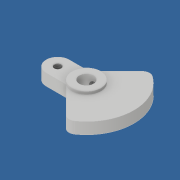
# Autodesk Inventor part: Kurbel 19
Saved by Autodesk Inventor 2018 (Build 220112000, 112)
## iProperties
Created: 2018-10-20
Part Number: Kurbel 19
Material: Generisch
Document SubType Name: Modeling
Designer: M.Knabel
Density: 1 g/cm^3
Appearance: Vorgabe
Mass: 1.78961 g
Surface Area: 14.1512 cm^2
Volume: 1.78961 cm^3
Author: M.Knabel
Autodesk Inventor part; units mm, degrees
ref_plane "YZ Plane" through (0, 0, 0) normal (1, 0, 0) x (0, 1, 0)
ref_plane "XZ Plane" through (0, 0, 0) normal (0, 1, 0) x (-1, 0, 0)
ref_plane "XY Plane" through (0, 0, 0) normal (0, 0, 1) x (1, 0, 0)
sketch "Skizze1" plane through (0, 0, 0) normal (0, 0, 1) x (1, 0, 0)
  line L0 (0, -20.5159) -> (0, 20.5159) projected
  line L1 (-20.1, 0) -> (22.6, 0) projected
  circle A0 centre (0, 0) radius 2.5
  arc A1 (-3, 4) -> (-3, -4) centre (0, 0) ccw
  arc A2 (7.5831, -14.6542) -> (7.5831, 14.6542) centre (0, 0) ccw
  line L2 (-3.5355, 3.5355) -> (7.5831, 14.6542)
  line L3 (-3.5355, -3.5355) -> (7.5831, -14.6542)
  line L4 (-3, 4) -> (-10, 4)
  line L5 (-3, -4) -> (-10, -4)
  arc A3 (-10, 4) -> (-10, -4) centre (-10, 0) ccw
  dimension "d0" = 5
  dimension "d1" = 10
  dimension "d3" = 33
  dimension "d4" = 90
  dimension "d5" = 4
  dimension "d6" = 10
  constraints: 8 end point, 8 point on circle, 4 centre point, 3 coincident, 3 tangent, 1 horizontal, 1 parallel, 1 point on line, 1 symmetric about line, 1 other
  measures "d0" diameter of A0
  measures "d1" diameter of A1
  measures "d3" diameter of A2
  measures "d4" angle of L3 L2
  measures "d5" radius of A3
  measures "d6" distance of A3.centre point (0, 0)
extrude "Extrusion1" add sketch "Skizze1" along normal blind 4 contours L3 L5 A1 L1 A0 L0 | L0 A0 L1 A2 L3 | L5 A3 L1 A1 L3 | L3 A1 L5 | L1 A1 L4 L2 L0 A0 | A0 L0 L2 A2 L1 | L1 A3 L4 L2 A1 | L2 L4 A1
fillet "Rundung1" radius 2.5 2 edges at (7.5831, 14.6542, 2) (7.5831, -14.6542, 2)
sketch "Skizze2" plane through (0, 0, 4) normal (0, 0, 1) x (1, 0, 0)
  arc A0 (-10, 4) -> (-10, -4) centre (-10, 0) ccw projected
  line L0 (0, -20.5159) -> (0, 20.5159) projected
  point P0 (0, 0)
  constraints: 1 coincident
hole "Bohrung1" at (-10, 0, 4) direction (0, 0, -1) diameter 2.459 end through all thread size "M3x0.5" class "6H" standard "ISO Metric profile"
sketch "Skizze3" plane through (0, 0, 4) normal (0, 0, 1) x (1, 0, 0)
  line L0 (0, -20.5159) -> (0, 20.5159) projected
  line L1 (-20.1, 0) -> (22.6, 0) projected
  line L2 (-10, -4) -> (-3.0711, -4) projected
  circle A0 centre (0, 0) radius 5.043
  circle A1 centre (0, 0) radius 2.5
  dimension "d17" = 5
  constraints: 2 coincident, 1 centre point, 3 other
  measures "d17" diameter of A1
extrude "Extrusion2" add sketch "Skizze3" along normal blind 1 contours A0 L1 A1 L0 | L0 A1 L1 A0 | L1 A1 L0 A0 | L1 A0 L0 A1
ref_plane "Arbeitsebene1" through (0, 10, 0) normal (0, 1, 0) x (-1, 0, 0)
sketch "Skizze7" plane through (0, 10, 0) normal (0, 1, 0) x (-1, 0, 0)
  line L0 (0, -0.8) -> (0, 4.8) projected
  line L1 (15, 0) -> (-2.5, 0) projected
  line L2 (10, 0) -> (10, 4) projected
  point P0 (0, 0)
  point P1 (0, 2)
  dimension "d30" = 2
  constraints: 1 midpoint
  measures "d30" distance from line of point (0, 2) L1
hole "Bohrung3" at (0, 10, 2) direction (0, -1, 0) diameter 3.5 depth 4.6
sketch "Skizze8" plane through (0, 5.4, 2) normal (0, 1, 0) x (1, 0, 0)
  line L0 (0, 3) -> (0, -4) projected
  line L1 (22.6, 2) -> (-20.1, 2) projected
  point P0 (0, 2)
  point P1 (0, 0)
  dimension "d38" = 2
  constraints: 1 point on line
  measures "d38" distance from line of point (0, 0) L1
hole "Bohrung4" at (0, 5.4, 2) direction (0, -1, 0) diameter 2.459 end up to face face through (0, 0, 0) facing (0, 0, 1) round with radius 2.5 far side yes thread size "M3x0.5" class "6H" standard "ISO Metric profile"
